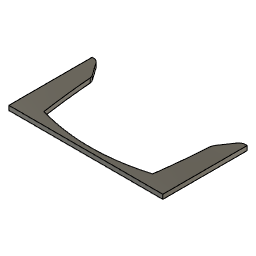
Top_Dispensor_holder (Autodesk Fusion 360 design; units mm, degrees)
Autodesk Fusion 360 part; units mm, degrees
sketch "Sketch1" plane through (0, 0, 0) normal (0, 0, 1) x (1, 0, 0)
  line L0 (0, 0) -> (70, 0)
  line L1 (70, 0) -> (70, 70)
  line L2 (70, 70) -> (0, 70)
  line L3 (0, 70) -> (0, 0)
  line L4 (35, 0) -> (35, 2)
  line L5 (7.0862, 38.0966) -> (-0.0002, 37.8975)
  spline S0 degree 3 poles (10.3955, 5.5731) (10.3802, 5.6793) (10.3649, 5.7855) (10.3496, 5.8917) (9.0883, 14.6436) (8.1004, 23.4498) (7.4637, 32.2724) (7.3237, 34.2127) (7.1982, 36.1541) (7.0862, 38.0966) knots -0.009814 -0.009814 -0.009814 -0.009814 0 0 0 0.807859 0.807859 0.807859 0.985531 0.985531 0.985531 0.985531
  spline S1 degree 3 poles (10.3955, 5.5731) (10.4984, 5.5428) (10.6014, 5.5124) (10.7043, 5.4821) (20.4404, 2.6148) (30.6917, 1.4904) (40.8231, 2.2123) (47.1025, 2.6598) (53.3356, 3.8196) (59.3506, 5.6366) (59.4527, 5.6674) (59.5548, 5.6983) (59.6569, 5.7291) knots -0.006564 -0.006564 -0.006564 -0.006564 0 0 0 0.617362 0.617362 0.617362 1 1 1 1.006532 1.006532 1.006532 1.006532
  spline S2 degree 3 poles (59.6569, 5.7291) (59.6713, 5.8348) (59.6858, 5.9405) (59.7002, 6.0462) (59.8076, 6.8337) (59.9283, 7.7587) (60.0441, 8.6669) (60.1266, 9.3143) (60.1999, 9.8958) (60.2654, 10.4307) (60.3347, 10.9971) (60.4027, 11.5764) (60.5122, 12.5559) (60.6287, 13.5983) (60.7932, 15.1018) (60.9645, 16.7322) (61.1308, 18.3151) (61.2956, 19.9486) (61.4243, 21.3369) (61.6198, 23.4449) (61.7373, 25.0266) (61.8616, 26.7626) (61.984, 28.4714) (62.1188, 30.3815) (62.2431, 32.3181) (62.3758, 34.386) (62.4877, 36.4096) (62.5659, 38.2906) knots -0.017354 -0.017354 -0.017354 -0.017354 0 0 0 0.129003 0.129003 0.129003 0.22097 0.22097 0.22097 0.318349 0.318349 0.318349 0.421987 0.421987 0.421987 0.522602 0.522602 0.522602 0.675374 0.675374 0.675374 0.825748 0.825748 0.825748 0.986316 0.986316 0.986316 0.986316
  line L6 (62.5659, 38.2906) -> (70, 38.3506)
  line L7 (10.3955, 5.5731) -> (10.3955, 0)
  line L8 (59.6569, 5.7291) -> (59.6569, 0)
  dimension "d2" = 70
  dimension "d3" = 70
  dimension "d4" = 2
  constraint horizontal L0
  constraint vertical L1
  constraint horizontal L2
  constraint vertical L3
  constraint coincident L0.start L3.end
  constraint midpoint L0 L4.start
  constraint perpendicular L0 L4
  constraint coincident L0 L7.end
  constraint perpendicular L0 L7
  constraint coincident L0 L8.end
  constraint perpendicular L0 L8
  constraint coincident L4.end S1
  measures "d2" distance of L0.start L0.end
  measures "d3" distance of L0.start L2.end
  measures "d4" distance of L4.start L4.end
extrude "Extrude1" add sketch "Sketch1" along normal blind 2 contours L0 L3 L5 S0 L7 | L0 L4 S1 L7 | L0 L4 S1 L8 | L0 L1 S2 L6 L8
chamfer "Chamfer2" distance 5 distance2 8 1 edges at (62.5659, 38.2906, 1) measured on face at (65.0439, 38.3106, 0.6667)
chamfer "Chamfer2" distance 8 distance2 5 1 edges at (7.0862, 38.0966, 1) measured on face at (9.6377, 11.0613, 0.6667)
fillet "Fillet3" radius 3 4 edges at (67.5657, 38.3309, 1) (62.1098, 30.3036, 1) (7.6264, 30.1149, 1) (2.0882, 37.9562, 1)
equation "Box_width = 70 mm"
equation "d2 = Box_width"
equation "d3 = Box_width"
